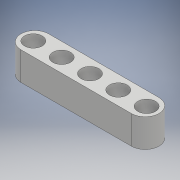
# Autodesk Inventor part: Transmission_Holder_5_Place_Holder
Saved by Autodesk Inventor 2018.2 (Build 222227000, 227)
## iProperties
Created: 2018-08-11
Part Number: Transmission_Holder_5_Place_Holder
Material: Generic
Document SubType Name: Modeling
Designer: mateu
Density: 1 g/cm^3
Appearance: Default
Author: mateu
Autodesk Inventor part; units mm, degrees
ref_plane "YZ Plane" through (0, 0, 0) normal (1, 0, 0) x (0, 1, 0)
ref_plane "XZ Plane" through (0, 0, 0) normal (0, 1, 0) x (-1, 0, 0)
ref_plane "XY Plane" through (0, 0, 0) normal (0, 0, 1) x (1, 0, 0)
sketch "Sketch1" plane through (0, 0, 0) normal (0, 0, 1) x (1, 0, 0)
  line L0 (0, 0) -> (39, 0)
  line L1 (39, 0) -> (39, -7.8)
  line L2 (39, -7.8) -> (0, -7.8)
  line L3 (0, -7.8) -> (0, 0)
  dimension "d0" = 39
  dimension "d1" = 7.8
  constraints: 8 end point, 2 parallel, 1 horizontal, 1 perpendicular
  measures "d0" distance of L1.end L2.end
  measures "d1" distance of L0.end L1.end
extrude "Extrusion1" add sketch "Sketch1" along normal blind 8
fillet "Fillet1" radius 3.9 1 edges at (0, 0, 4)
fillet "Fillet2" radius 3.9 1 edges at (0, -7.8, 4)
fillet "Fillet3" radius 3.9 1 edges at (39, -7.8, 4)
fillet "Fillet4" radius 3.9 1 edges at (39, 0, 4)
sketch "Sketch2" plane through (0, 0, 8) normal (0, 0, 1) x (1, 0, 0)
  line L0 (35.1, 0) -> (3.9, 0) projected
  arc A0 (35.1, -7.8) -> (35.1, 0) centre (35.1, -3.9) ccw projected
  line L1 (0, -3.9) -> (39, -3.9)
  circle A1 centre (19.5, -3.9) radius 2.5
  circle A2 centre (27.5, -3.9) radius 2.5
  circle A3 centre (35.5, -3.9) radius 2.5
  circle A4 centre (11.5, -3.9) radius 2.5
  circle A5 centre (3.5, -3.9) radius 2.5
  point P0 (0, 0)
  dimension "d16" = 39
  dimension "d17" = 5
  dimension "d18" = 5
  dimension "d19" = 5
  dimension "d20" = 5
  dimension "d21" = 5
  dimension "d24" = 3
  dimension "d25" = 3
  dimension "d27" = 3
  dimension "d28" = 3
  constraints: 5 centre point, 4 point on line, 2 end point, 1 midpoint, 1 point on circle
  measures "d16" distance of L1.start L1.end
  measures "d17" diameter of A1
  measures "d18" diameter of A2
  measures "d19" diameter of A3
  measures "d20" diameter of A4
  measures "d21" diameter of A5
extrude "Extrusion2" cut sketch "Sketch2" against normal blind 8
body "Solid1"
